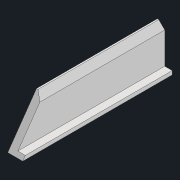
# Autodesk Inventor part: s_base4
Saved by Autodesk Inventor 2021 (Build 250183000, 183)
## iProperties
Created: 2021-08-20
Part Number: s_base4
Material: 一般
Document SubType Name: Modeling
Designer: yuta0
Density: 1 g/cm^3
Appearance: 既定
Author: yuta0
Autodesk Inventor part; units mm, degrees
ref_plane "YZ Plane" through (0, 0, 0) normal (1, 0, 0) x (0, 1, 0)
ref_plane "XZ Plane" through (0, 0, 0) normal (0, 1, 0) x (-1, 0, 0)
ref_plane "XY Plane" through (0, 0, 0) normal (0, 0, 1) x (1, 0, 0)
sketch "スケッチ1" plane through (0, 0, 0) normal (0, 0, 1) x (1, 0, 0)
  line L0 (-20, -2.5) -> (20, -2.5)
  line L1 (20, -2.5) -> (20, 2.5)
  line L2 (-20, 2.5) -> (-20, -2.5)
  line L3 (-20, -2.5) -> (20, 2.5) construction
  line L4 (20, -2.5) -> (-20, 2.5) construction
  line L5 (-10, 2.5) -> (10, 2.5)
  line L6 (10, 2.5) -> (10, 33.5)
  line L7 (10, 33.5) -> (-10, 33.5)
  line L8 (-10, 33.5) -> (-10, 2.5)
  line L9 (-10, 2.5) -> (10, 33.5) construction
  line L10 (10, 2.5) -> (-10, 33.5) construction
  line L11 (20, 2.5) -> (10, 2.5)
  line L12 (-10, 2.5) -> (-20, 2.5)
  line L13 (0, 33.5) -> (0, -2.5)
  point P0 (0, 0)
  point P1 (0, 18)
  point P2 (0, 18)
  point P3 (0, 0)
  dimension "d0" = 20
  dimension "d1" = 31
  dimension "d2" = 5
  dimension "d3" = 10
  constraints: 28 end point, 8 midpoint, 5 parallel, 2 horizontal, 2 perpendicular, 1 vertical alignment
  measures "d0" distance of L6.end L7.end
  measures "d1" distance of L5.end L6.end
  measures "d2" distance of L0.end L1.end
  measures "d3" distance between parallel lines of L8 L2
extrude "押し出し1" add sketch "スケッチ1" along normal mid plane 200 contours L13 L5 L11 L1 L0 | L13 L7 L6 L5
sketch "スケッチ4" plane through (0, -2.5, 100) normal (-1, 0, 0) x (0, 0, 1)
  line L0 (0, 0) -> (-25.2075, 36)
  line L1 (-200, 36) -> (0, 36) projected
  line L2 (0, 36) -> (0, 0) projected
  point P0 (-100, 2.5)
  dimension "d18" = 35
  constraints: 2 end point, 1 coincident, 1 point on line
  measures "d18" angle of L2 L0
extrude "押し出し3" cut sketch "スケッチ4" against normal through all
